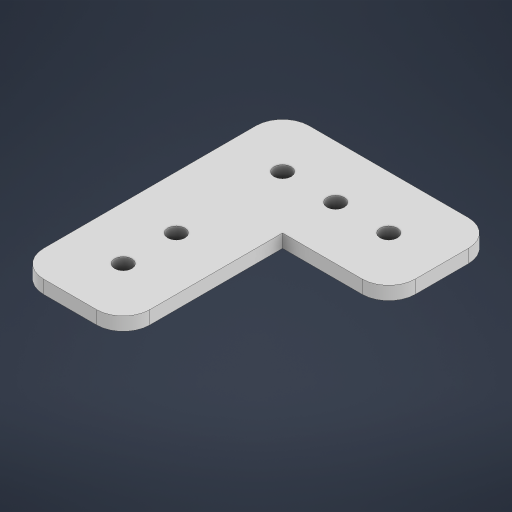
# Autodesk Inventor part: fram_support_gusset
Saved by Autodesk Inventor 2023 (Build 270158000, 158)
## iProperties
Created: 2023-02-13
Part Number: fram_support_gusset
Material: Generic
Document SubType Name: Modeling
Designer: bryce
Density: 1 g/cm^3
Appearance: Default
Author: bryce
Autodesk Inventor part; units mm, degrees
ref_plane "YZ Plane" through (0, 0, 0) normal (1, 0, 0) x (0, 1, 0)
ref_plane "XZ Plane" through (0, 0, 0) normal (0, 1, 0) x (-1, 0, 0)
ref_plane "XY Plane" through (0, 0, 0) normal (0, 0, 1) x (1, 0, 0)
sketch "Sketch1" plane through (0, 0, 0) normal (0, 1, 0) x (-1, 0, 0)
  line L0 (0, 0) -> (-50.8, 0)
  line L1 (-50.8, 0) -> (-50.8, -63.5)
  line L2 (-50.8, -63.5) -> (0, -63.5)
  line L3 (0, -63.5) -> (0, 0)
  line L4 (-50.8, -63.5) -> (-50.8, -38.1)
  line L5 (-50.8, -38.1) -> (-25.4, -38.1)
  line L6 (-25.4, -38.1) -> (-25.4, 0)
  circle A0 centre (-25.4, -50.8) radius 2.0638
  line L7 (-50.8, -50.8) -> (0, -50.8) construction
  circle A1 centre (-38.1, -50.8) radius 2.0637
  circle A2 centre (-12.7, -50.8) radius 2.0637
  line L8 (-12.7, -63.5) -> (-12.7, 0) construction
  circle A3 centre (-12.7, -25.4) radius 2.0638
  circle A4 centre (-12.7, -12.7) radius 2.0638
  dimension "d22" = 50.8
  dimension "d23" = 63.5
  dimension "d24" = 25.4
  dimension "d25" = 25.4
  dimension "d26" = 4.1275
  dimension "d27" = 4.1275
  dimension "d28" = 12.7
  dimension "d29" = 4.1275
  dimension "d30" = 12.7
  dimension "d31" = 4.1275
  dimension "d32" = 25.4
  dimension "d33" = 4.1275
  dimension "d34" = 12.7
  constraints: 18 end point, 8 point on line, 5 centre point, 3 midpoint, 3 perpendicular, 2 horizontal, 2 parallel
  measures "d22" distance of L2.end L1.end
  measures "d23" distance of L1.end L0.end
  measures "d24" distance of L1.end L4.end
  measures "d25" distance of L4.end L5.end
  measures "d26" diameter of A0
  measures "d27" diameter of A1
  measures "d28" distance of L7.start A1.centre
  measures "d29" diameter of A2
  measures "d30" distance of point (-25.4, -50.8) A2.centre
  measures "d31" diameter of A3
  measures "d32" distance of A2.centre A3.centre
  measures "d33" diameter of A4
  measures "d34" distance of A3.centre A4.centre
extrude "Extrusion1" add sketch "Sketch1" along normal blind 3.175 contours L3 L2 L1 L5 L6 L0
fillet "Fillet1" radius 6.35 5 edges at (50.8, 1.5875, -38.1) (25.4, 1.5875, 0) (0, 1.5875, 0) (0, 1.5875, -63.5) (50.8, 1.5875, -63.5)
body "Solid1"
